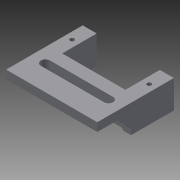
# Autodesk Inventor part: servolock1
Saved by Autodesk Inventor 2015 (Build 190159000, 159)
## iProperties
Created: 2020-08-08
Part Number: servolock1
Material: 일반
Document SubType Name: Modeling
Designer: penta
Density: 1 g/cm^3
Appearance: 기본값
Author: penta
Autodesk Inventor part; units mm, degrees
ref_plane "YZ Plane" through (0, 0, 0) normal (1, 0, 0) x (0, 1, 0)
ref_plane "XZ Plane" through (0, 0, 0) normal (0, 1, 0) x (-1, 0, 0)
ref_plane "XY Plane" through (0, 0, 0) normal (0, 0, 1) x (1, 0, 0)
sketch "스케치1" plane through (0, 0, 0) normal (0, 0, 1) x (1, 0, 0)
  line L0 (0, 0) -> (22.5, 0)
  line L1 (22.5, 0) -> (22.5, 12.3)
  line L2 (0, 12.3) -> (0, 0)
  line L3 (-5, -3) -> (27.5, -3)
  line L4 (27.5, -3) -> (27.5, 12.3)
  line L5 (27.5, 12.3) -> (22.5, 12.3)
  line L6 (-5, 12.3) -> (-5, -3)
  line L7 (0, 12.3) -> (-5, 12.3)
  dimension "d0" = 22.5
  dimension "d1" = 12.3
  dimension "d2" = 32.5
  constraints: 16 end point, 4 parallel, 2 horizontal, 2 perpendicular
  measures "d0" distance of L2.start L1.end
  measures "d1" distance of L1.end L0.end
  measures "d2" distance of L6.start L4.end
extrude "돌출1" add sketch "스케치1" against normal blind 10
hole "구멍1" at (25, 6, 0) direction (0, 0, -1) diameter 1.5 depth 10 tip angle 118
hole "구멍2" at (-2.5, 6, 0) direction (0, 0, -1) diameter 1.5 depth 10 tip angle 118
sketch "스케치3" plane through (-5, -3, 0) normal (0, -1, 0) x (1, 0, 0)
  line L0 (32.5, 0) -> (32.5, -10) projected
  line L1 (0, 0) -> (32.5, 0)
  line L2 (32.5, 0) -> (32.5, -3)
  line L3 (32.5, -3) -> (0, -3)
  line L4 (0, -3) -> (0, 0)
  point P0 (5, 0)
  point P1 (32.5, -13)
  dimension "d34" = 3
  constraints: 8 end point, 2 parallel, 1 horizontal, 1 perpendicular, 1 point on line
  measures "d34" distance of L1.end L2.end
extrude "돌출3" add sketch "스케치3" along normal blind 12
sketch "스케치4" plane through (27.5, -3, -3) normal (0, 0, -1) x (-1, 0, 0)
  line L0 (27.5, -3) -> (5, -3) construction
  line L1 (27.5, -1.375) -> (5, -1.375)
  line L2 (5, -4.625) -> (27.5, -4.625)
  arc A0 (27.5, -4.625) -> (27.5, -1.375) centre (27.5, -3) ccw
  arc A1 (5, -1.375) -> (5, -4.625) centre (5, -3) ccw
  point P0 (27.5, 3)
  point P1 (16.25, -3)
  dimension "d38" = 22.5
  dimension "d39" = 3.25
  constraints: 8 end point, 4 point on circle, 4 tangent, 2 centre point, 1 horizontal, 1 midpoint, 1 parallel
  measures "d38" distance of L0.start L0.end
  measures "d39" diameter of A1
extrude "돌출4" cut sketch "스케치4" against normal through all
sketch "스케치5" plane through (0, 0, -10) normal (0, 0, -1) x (-1, 0, 0)
  arc A0 (-22.5, -4.375) -> (-22.5, -7.625) centre (-22.5, -6) ccw projected
  line L0 (-22.5, -4.375) -> (0, -4.375) projected
  line L1 (0, -7.625) -> (-22.5, -7.625) projected
  arc A1 (0, -7.625) -> (0, -4.375) centre (0, -6) ccw projected
  line L2 (-22.5, -6) -> (0, -6) construction
  line L3 (-22.5, -9.75) -> (0, -9.75)
  line L4 (0, -2.25) -> (-22.5, -2.25)
  arc A2 (-22.5, -2.25) -> (-22.5, -9.75) centre (-22.5, -6) ccw
  arc A3 (0, -9.75) -> (0, -2.25) centre (0, -6) ccw
  point P0 (0, 0)
  point P1 (-11.25, -6)
  dimension "d40" = 7.5
  constraints: 8 end point, 4 point on circle, 4 tangent, 2 centre point, 1 horizontal, 1 midpoint, 1 parallel
  measures "d40" diameter of A3
extrude "돌출5" cut sketch "스케치5" against normal up to surface (7 mm away) contours L0 A1 L1 A0 | A2 L4 A3 L3
chamfer "모따기1" distance 5 angle 45 2 edges at (-3.625, -3, -3) (26.125, -3, -3)
